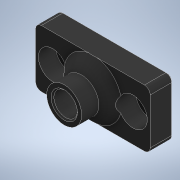
# Autodesk Inventor part: RodHolder_1
Saved by Autodesk Inventor 2021 (Build 250183000, 183)
## iProperties
Created: 2020-07-16
Part Number: RodHolder_1
Material: Generic
Document SubType Name: Modeling
Designer: CASE-SMALL2
Density: 1 g/cm^3
Appearance: Default
Author: CASE-SMALL2
## iProperties of the stored document _3DPrint.ipt
Created: 2020-07-17
Part Number: _3DPrint
Material: Generic
Document SubType Name: Modeling
Designer: CASE-SMALL2
Density: 1 g/cm^3
Appearance: Default
Author: CASE-SMALL2
Autodesk Inventor part; units mm, degrees
ref_plane "YZ Plane" through (0, 0, 0) normal (1, 0, 0) x (0, 1, 0)
ref_plane "XZ Plane" through (0, 0, 0) normal (0, 1, 0) x (-1, 0, 0)
ref_plane "XY Plane" through (0, 0, 0) normal (0, 0, 1) x (1, 0, 0)
sketch "Sketch1" plane through (0, 0, 0) normal (0, 0, 1) x (1, 0, 0)
  line L0 (-20, -10) -> (20, -10)
  line L1 (20, -10) -> (20, 10)
  line L2 (20, 10) -> (-20, 10)
  line L3 (-20, 10) -> (-20, -10)
  line L4 (-20, -10) -> (20, 10) construction
  line L5 (20, -10) -> (-20, 10) construction
  line L6 (-28, 0) -> (28, 0) projected
  circle A0 centre (-14, 0) radius 2.4
  circle A1 centre (14, 0) radius 2.4
  point P0 (0, 0)
  dimension "d0" = 40
  dimension "d1" = 20
  dimension "d2" = 4.8
  dimension "d3" = 4.8
  dimension "d4" = 6
  dimension "d5" = 6
  constraints: 12 end point, 2 centre point, 2 midpoint, 2 parallel, 2 point on line, 1 horizontal, 1 perpendicular
  measures "d0" distance of L1.end L2.end
  measures "d1" distance of L0.end L1.end
  measures "d2" diameter of A0
  measures "d3" diameter of A1
  measures "d4" distance from line of L3 A0.centre
  measures "d5" distance from line of L1 A1.centre
extrude "Extrusion1" add sketch "Sketch1" along normal blind 8 contours L3 L6 A0 A1 L1 L0 | L3 L2 L1 L6 A1 A0
fillet "Fillet1" radius 2 4 edges at (20, -10, 4) (20, 10, 4) (-20, 10, 4) (-20, -10, 4)
sketch "Sketch2" plane through (0, 0, 8) normal (0, 0, 1) x (1, 0, 0)
  circle A0 centre (0, 0) radius 4.1
  circle A1 centre (0, 0) radius 6.1
  dimension "d9" = 8.2
  dimension "d24" = 2
  constraints: 2 centre point, 2 coincident
  measures "d9" diameter of A0
  measures "d24" radial gap between concentric circles of A1 A0
extrude "Extrusion2" add sketch "Sketch2" along normal blind 10
chamfer "Chamfer1" distance 4 angle 45 1 edges at (-6.1, 0, 8)
chamfer "Chamfer2" distance 0.5 angle 45 1 edges at (-4.1, 0, 18)
sketch "Sketch5" plane through (0, 0, 8) normal (0, 0, 1) x (1, 0, 0)
  circle A0 centre (-14, 0) radius 2.4 projected
  line L0 (-28, 0) -> (28, 0) construction
  line L1 (0, -14) -> (0, 14) projected
  circle A1 centre (-14, 0) radius 5
  circle A2 centre (14, 0) radius 2.4
  circle A3 centre (14, 0) radius 5
  point P0 (0, 0)
  dimension "d28" = 10
  constraints: 3 centre point, 2 coincident, 2 symmetric about line, 2 other
  measures "d28" diameter of A1
extrude "Extrusion4" cut sketch "Sketch5" along normal blind 8
sketch "Sketch6" plane through (0, 0, 8) normal (0, 0, 1) x (1, 0, 0)
  circle A0 centre (14, 0) radius 2.4 projected
  circle A1 centre (-14, 0) radius 2.4 projected
  circle A2 centre (14, 0) radius 5
  circle A3 centre (-14, 0) radius 5
  point P0 (0, 0)
  dimension "d31" = 10
  dimension "d32" = 10
  constraints: 2 centre point, 2 coincident
  measures "d31" diameter of A2
  measures "d32" diameter of A3
extrude "Extrusion5" cut sketch "Sketch6" against normal blind 6
chamfer "Chamfer3" distance 0.5 angle 45 8 edges at (0, -10, 0) (19.4142, -9.4142, 0) (20, 0, 0) (19.4142, 9.4142, 0) (0, 10, 0) (-19.4142, 9.4142, 0) (-20, 0, 0) (-19.4142, -9.4142, 0)
equation "\"d3\" = d2"
equation "\"d5\" = d4"
equation "\"d32\" = d31"
body "Solid1"
